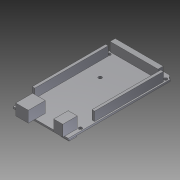
# Autodesk Inventor part: Arduino
Saved by Autodesk Inventor 2011 SP2 (Build 150309200, 309)
## iProperties
Created: 2015-01-24
Part Number: Arduino
Document SubType Name: Modeling
Designer: Ernest
Density: 1 g/cm^3
Mass: 15.9204 g
Surface Area: 125.226 cm^2
Volume: 15.9204 cm^3
Author: Ernest
Autodesk Inventor part; units mm, degrees
ref_plane "YZ Plane" through (0, 0, 0) normal (1, 0, 0) x (0, 1, 0)
ref_plane "XZ Plane" through (0, 0, 0) normal (0, 1, 0) x (-1, 0, 0)
ref_plane "XY Plane" through (0, 0, 0) normal (0, 0, 1) x (1, 0, 0)
sketch "Sketch1" plane through (0, 0, 0) normal (0, 0, 1) x (1, 0, 0)
  line L0 (0, 0) -> (102, 0)
  line L1 (102, 0) -> (102, 1.7)
  line L2 (102, 1.7) -> (0, 1.7)
  line L3 (0, 1.7) -> (0, 0)
  dimension "d0" = 102
  dimension "d1" = 1.7
  constraints: 8 end point, 2 parallel, 1 horizontal, 1 perpendicular
  measures "d0" distance of L2.end L1.end
  measures "d1" distance between parallel lines of L0 L2
extrude "Extrusion1" add sketch "Sketch1" along normal blind 53.3
sketch "Sketch3" plane through (0, 1.7, 53.3) normal (0, 1, 0) x (1, 0, 0)
  line L0 (102, 53.3) -> (0, 53.3) projected
  line L1 (0, 53.3) -> (0, 0) projected
  line L2 (0, 0) -> (102, 0) projected
  line L3 (9.75, 44.2) -> (-6.65, 44.2)
  line L4 (-6.65, 44.2) -> (-6.65, 32)
  line L5 (-6.65, 32) -> (9.75, 32)
  line L6 (9.75, 32) -> (9.75, 44.2)
  line L7 (12.3, 12.4) -> (-1.7, 12.4)
  line L8 (-1.7, 12.4) -> (-1.7, 3.6)
  line L9 (-1.7, 3.6) -> (12.3, 3.6)
  line L10 (12.3, 3.6) -> (12.3, 12.4)
  line L11 (102, 0) -> (0, 0) projected
  line L12 (99, 0) -> (99, 1.4)
  line L13 (99, 1.4) -> (102, 4)
  line L14 (102, 4) -> (102, 39.12)
  line L15 (102, 53.3) -> (102, 0) projected
  line L16 (102, 39.12) -> (98.6, 41.3)
  line L17 (98.6, 41.3) -> (98.6, 50.3)
  line L18 (98.6, 50.3) -> (95.6, 53.3)
  line L19 (0, 53.3) -> (102, 53.3) projected
  circle A0 centre (96.75, 2.55) radius 1.65
  circle A1 centre (90.05, 50.75) radius 1.65
  circle A2 centre (66.35, 35.45) radius 1.65
  circle A3 centre (66.35, 7.65) radius 1.65
  circle A4 centre (15.25, 50.75) radius 1.65
  circle A5 centre (14.25, 2.55) radius 1.65
  line L20 (88.15, 49.5) -> (17.15, 49.5)
  line L21 (17.15, 49.5) -> (17.15, 52)
  line L22 (17.15, 52) -> (88.15, 52)
  line L23 (88.15, 52) -> (88.15, 49.5)
  line L24 (93.3, 1.3) -> (26.8, 1.3)
  line L25 (26.8, 1.3) -> (26.8, 3.8)
  line L26 (26.8, 3.8) -> (93.3, 3.8)
  line L27 (93.3, 3.8) -> (93.3, 1.3)
  line L28 (97.65, 52.2) -> (92.65, 52.2)
  line L29 (92.65, 52.2) -> (92.65, 5.8)
  line L30 (92.65, 5.8) -> (97.65, 5.8)
  line L31 (97.65, 5.8) -> (97.65, 52.2)
  dimension "d23" = 9.1
  dimension "d24" = 9.75
  dimension "d25" = 16.4
  dimension "d26" = 12.2
  dimension "d27" = 8.8
  dimension "d28" = 14
  dimension "d29" = 12.4
  dimension "d30" = 1.7
  dimension "d44" = 3
  dimension "d45" = 3.4
  dimension "d46" = 3
  dimension "d47" = 3
  dimension "d48" = 1.4
  dimension "d49" = 4
  dimension "d50" = 35.12
  dimension "d51" = 12
  dimension "d52" = 3.3
  dimension "d53" = 3.3
  dimension "d54" = 3.3
  dimension "d55" = 3.3
  dimension "d56" = 3.3
  dimension "d57" = 3.3
  dimension "d58" = 0.9
  dimension "d59" = 3.6
  dimension "d60" = 6.9
  dimension "d61" = 0.9
  dimension "d62" = 0.9
  dimension "d63" = 0.9
  dimension "d64" = 13.6
  dimension "d66" = 12.6
  dimension "d67" = 34
  dimension "d69" = 34
  dimension "d70" = 6
  dimension "d71" = 16.2
  dimension "d72" = 71
  dimension "d73" = 0.25
  dimension "d74" = 2.5
  dimension "d75" = 1.25
  dimension "d76" = 66.5
  dimension "d77" = 2.5
  dimension "d78" = 1.25
  dimension "d79" = 1.8
  dimension "d80" = 5
  dimension "d81" = 46.4
  dimension "d82" = 1.1
  dimension "d83" = 0.95
  constraints: 52 end point, 11 parallel, 6 centre point, 6 perpendicular, 5 horizontal, 3 point on line
  measures "d23" distance between parallel lines of L3 L0
  measures "d24" distance between parallel lines of L6 L1
  measures "d25" distance of L4.end L5.end
  measures "d26" distance of L5.end L3.start
  measures "d27" distance of L7.end L8.end
  measures "d28" distance of L7.start L7.end
  measures "d29" distance between parallel lines of L2 L7
  measures "d30" distance between parallel lines of L1 L8
  measures "d44" distance from line of L14 L12.start
  measures "d45" distance between parallel lines of L14 L17
  measures "d46" distance from line of L17 L18.end
  measures "d47" distance from line of L0 L17.end
  measures "d48" distance of L12.start L12.end
  measures "d49" vertical distance of L13.end L12.start
  measures "d50" distance of L13.end L14.end
  measures "d51" vertical distance of L18.end L16.end
  measures "d52" diameter of A0
  measures "d53" diameter of A3
  measures "d54" diameter of A5
  measures "d55" diameter of A2
  measures "d56" diameter of A1
  measures "d57" diameter of A4
  measures "d58" distance edge to line of A0 L11
  measures "d59" distance edge to line of A0 L15
  measures "d60" distance edge to line of A1 L17
  measures "d61" distance edge to line of A1 L0
  measures "d62" distance edge to line of A4 L0
  measures "d63" distance edge to line of A5 L11
  measures "d64" distance edge to line of A4 L1
  measures "d66" distance edge to line of A5 L1
  measures "d67" distance edge to line of A2 L14
  measures "d69" distance edge to line of A3 L15
  measures "d70" distance edge to line of A3 L2
  measures "d71" distance edge to line of A2 L0
  measures "d72" distance of L21.end L22.end
  measures "d73" distance edge to line of A1 L23
  measures "d74" distance between parallel lines of L22 L20
  measures "d75" distance from line of A1.centre L20
  measures "d76" distance of L25.end L26.end
  measures "d77" distance between parallel lines of L26 L24
  measures "d78" distance from line of A0.centre L24
  measures "d79" distance edge to line of A0 L27
  measures "d80" distance of L30.end L29.end
  measures "d81" distance of L29.end L28.end
  measures "d82" distance between parallel lines of L19 L28
  measures "d83" distance between parallel lines of L17 L31
extrude "Extrusion3" add sketch "Sketch3" along normal blind 10.8 contours L3 L6 L5 L1 | L1 L5 L4 L3 | L7 L10 L9 L1 | L1 L9 L8 L7
extrude "Extrusion9" cut sketch "Sketch3" against normal blind 10 contours L15 L16 L17 L18 L31 L28 L0 | L28 L31 L18 | L15 L2 L12 L13 | A0 | A1 | A2 | A3 | A4 | A5
extrude "Extrusion10" add sketch "Sketch3" along normal blind 8.7 contours L28 L31 L18 | L18 L31 L30 L29 L28 | L20 L21 L22 L23 | L24 L25 L26 L27
sketch "Sketch7" plane through (0, 0, 0) normal (0, -1, 0) x (1, 0, 0)
  line L0 (26.8, 52) -> (26.8, 49.5) projected
  line L1 (93.3, 52) -> (26.8, 52) projected
  line L2 (93.3, 49.5) -> (93.3, 52) projected
  line L3 (26.8, 49.5) -> (93.3, 49.5) projected
  line L4 (17.15, 3.8) -> (17.15, 1.3) projected
  line L5 (88.15, 3.8) -> (17.15, 3.8) projected
  line L6 (88.15, 1.3) -> (88.15, 3.8) projected
  line L7 (17.15, 1.3) -> (88.15, 1.3) projected
  line L8 (97.65, 1.1) -> (97.65, 47.5) projected
  line L9 (92.65, 1.1) -> (97.65, 1.1) projected
  line L10 (92.65, 47.5) -> (92.65, 1.1) projected
  line L11 (97.65, 47.5) -> (92.65, 47.5) projected
  line L12 (87.5288, 2.0107) -> (17.9769, 2.0107)
  line L13 (17.9769, 2.0107) -> (17.9769, 3.0107)
  line L14 (17.9769, 3.0107) -> (87.5288, 3.0107)
  line L15 (87.5288, 3.0107) -> (87.5288, 2.0107)
  line L16 (92.4851, 50.2518) -> (27.6531, 50.2518)
  line L17 (27.6531, 50.2518) -> (27.6531, 51.2518)
  line L18 (27.6531, 51.2518) -> (92.4851, 51.2518)
  line L19 (92.4851, 51.2518) -> (92.4851, 50.2518)
  line L20 (96.9467, 2.0107) -> (95.9467, 2.0107)
  line L21 (95.9467, 2.0107) -> (95.9467, 46.8913)
  line L22 (95.9467, 46.8913) -> (96.9467, 46.8913)
  line L23 (96.9467, 46.8913) -> (96.9467, 2.0107)
  line L24 (93.4467, 46.8913) -> (94.4467, 46.8913)
  line L25 (94.4467, 46.8913) -> (94.4467, 2.0107)
  line L26 (94.4467, 2.0107) -> (93.4467, 2.0107)
  line L27 (93.4467, 2.0107) -> (93.4467, 46.8913)
  line L28 (12.3, 40.9) -> (12.3, 49.7) projected
  line L29 (-1.7, 40.9) -> (12.3, 40.9) projected
  line L30 (-1.7, 49.7) -> (-1.7, 40.9) projected
  line L31 (12.3, 49.7) -> (-1.7, 49.7) projected
  line L32 (9.75, 9.1) -> (9.75, 21.3) projected
  line L33 (-6.65, 9.1) -> (9.75, 9.1) projected
  line L34 (-6.65, 21.3) -> (-6.65, 9.1) projected
  line L35 (9.75, 21.3) -> (-6.65, 21.3) projected
  line L36 (0, 9.1) -> (9.75, 9.1) projected
  line L37 (6.6731, 6.8776) -> (3.1632, 6.8776)
  line L38 (3.1632, 6.8776) -> (3.1632, 9.1)
  line L39 (3.1632, 9.1) -> (6.6731, 9.1)
  line L40 (6.6731, 9.1) -> (6.6731, 6.8776)
  line L41 (9.75, 21.3) -> (0, 21.3) projected
  line L42 (6.6731, 21.3) -> (3.1632, 21.3)
  line L43 (3.1632, 21.3) -> (3.1632, 24.3)
  line L44 (3.1632, 24.3) -> (6.6731, 24.3)
  line L45 (6.6731, 24.3) -> (6.6731, 21.3)
  line L46 (9.75, 44) -> (2.1298, 44)
  line L47 (2.1298, 44) -> (2.1298, 51.9)
  line L48 (2.1298, 51.9) -> (9.75, 51.9)
  line L49 (9.75, 51.9) -> (9.75, 44)
  dimension "d110" = 1
  dimension "d111" = 1
  dimension "d112" = 1
  dimension "d113" = 1.5
  dimension "d114" = 1
  constraints: 56 end point, 14 parallel, 7 horizontal, 7 perpendicular, 2 point on line
  measures "d110" distance between parallel lines of L14 L12
  measures "d111" distance between parallel lines of L25 L27
  measures "d112" distance between parallel lines of L21 L23
  measures "d113" distance between parallel lines of L25 L21
  measures "d114" distance between parallel lines of L18 L16
extrude "Extrusion12" add sketch "Sketch7" along normal blind 1.3 contours L12 L13 L14 L15 | L16 L17 L18 L19 | L20 L21 L22 L23 | L24 L25 L26 L27
extrude "Extrusion13" add sketch "Sketch7" along normal blind 2.5 contours L49 L46 L47 L31 | L31 L47 L48 L49 | L40 L37 L38 L33 | L35 L43 L44 L45
body "Solid1"
